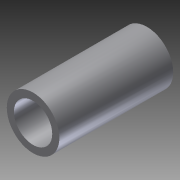
# Autodesk Inventor part: BatteryLatch-Spring
Saved by Autodesk Inventor 2012 (Build 160160000, 160)
## iProperties
Created: 2013-10-13
Part Number: BatteryLatch-Spring
Material: Default
Document SubType Name: Modeling
Designer: joe_000
Density: 1 g/cm^3
springDiameter: 0.375 in
springLength: 0.813 in
Author: joe_000
Autodesk Inventor part; units mm, degrees
ref_plane "YZ Plane" through (0, 0, 0) normal (1, 0, 0) x (0, 1, 0)
ref_plane "XZ Plane" through (0, 0, 0) normal (0, 1, 0) x (-1, 0, 0)
ref_plane "XY Plane" through (0, 0, 0) normal (0, 0, 1) x (1, 0, 0)
sketch "Sketch1" plane through (0, 0, 0) normal (0, 0, 1) x (1, 0, 0)
  circle A0 centre (0, 0) radius 4.7625
  circle A1 centre (0, 0) radius 3.4696
  dimension "springDiameter" = 9.525
  dimension "d3" = 6.9392
  constraints: 2 centre point, 2 coincident
  measures "springDiameter" diameter of A0
  measures "d3" diameter of A1
extrude "Extrusion1" add sketch "Sketch1" along normal blind 20.6375
body "Solid1"
